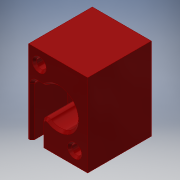
# Autodesk Inventor part: Base
Saved by Autodesk Inventor 2019 (Build 230136000, 136)
## iProperties
Created: 2021-01-03
Part Number: Base
Material: ABS Plastic
Document SubType Name: Modeling
Designer: Sam
Density: 1.06 g/cm^3
Appearance: Red
Author: Sam
Autodesk Inventor part; units mm, degrees
ref_plane "YZ Plane" through (0, 0, 0) normal (1, 0, 0) x (0, 1, 0)
ref_plane "XZ Plane" through (0, 0, 0) normal (0, 1, 0) x (-1, 0, 0)
ref_plane "XY Plane" through (0, 0, 0) normal (0, 0, 1) x (1, 0, 0)
sketch "Sketch1" plane through (0, 0, 0) normal (0, 0, 1) x (1, 0, 0)
  line L0 (12.5, 17.5) -> (-12.5, 17.5)
  line L1 (-12.5, 17.5) -> (-12.5, -17.5)
  line L2 (-12.5, -17.5) -> (12.5, -17.5)
  line L3 (12.5, -17.5) -> (12.5, 17.5)
  point P0 (0, 0)
  point P1 (12.5, 0)
  dimension "d0" = 25
  dimension "d1" = 35
  dimension "d16" = 12.5
  constraints: 8 end point, 2 parallel, 1 horizontal, 1 horizontal alignment, 1 midpoint, 1 perpendicular
  measures "d0" distance of L1.end L2.end
  measures "d1" distance of L2.end L0.start
  measures "d16" distance from line of point (0, 0) L3
extrude "Extrusion1" add sketch "Sketch1" along normal blind 12
sketch "Sketch2" plane through (0, 0, 12) normal (0, 0, 1) x (1, 0, 0)
  circle A0 centre (0, 0) radius 3.05
  dimension "d4" = 6.1
  constraints: 1 centre point, 1 coincident
  measures "d4" diameter of A0
extrude "Extrusion2" cut sketch "Sketch2" against normal up to next
sketch "Sketch4" plane through (0, 0, 12) normal (0, 0, 1) x (1, 0, 0)
  circle A0 centre (0, 0) radius 3.05 projected
  arc A1 (-7, -3.0859) -> (-5.7899, 5) centre (0, 0) ccw
  line L0 (-5.7899, 5) -> (-11, 5)
  line L1 (-11, 5) -> (-11, -17.5)
  line L2 (-12.5, -17.5) -> (12.5, -17.5) projected
  line L3 (-7, -3.0859) -> (-7, -17.5)
  circle A2 centre (0, 0) radius 3.05 projected
  line L4 (12.5, 17.5) -> (-12.5, 17.5) projected
  line L5 (-12.5, 17.5) -> (-12.5, -17.5) projected
  line L6 (-12.5, -17.5) -> (12.5, -17.5) projected
  line L7 (12.5, -17.5) -> (12.5, 17.5) projected
  dimension "d9" = 15.3
  dimension "d10" = 11
  dimension "d11" = 7
  dimension "d12" = 5
  constraints: 6 end point, 2 point on circle, 2 point on line, 1 centre point, 1 coincident, 1 horizontal, 1 parallel, 1 perpendicular
  measures "d9" diameter of A1
  measures "d10" distance from line of point (0, 0) L1
  measures "d11" distance from line of point (0, 0) L3
  measures "d12" distance from line of point (0, 0) L0
extrude "Extrusion3" add sketch "Sketch4" along normal blind 15 contours A1 L0 L1 L2 L5 L4 L7 L3
fillet "Fillet1" radius 2 3 edges at (-7, -3.0859, 19.5) (-5.7899, 5, 19.5) (-11, 5, 19.5)
sketch "Sketch5" plane through (0, 0, 27) normal (0, 0, 1) x (1, 0, 0)
  point P0 (0, 0)
  point P1 (-8, 12)
  point P2 (7, -12)
  dimension "d17" = 7
  dimension "d18" = 12
  dimension "d19" = 12
  dimension "d20" = 8
  measures "d17" horizontal distance of point (7, -12) point (0, 0)
  measures "d18" vertical distance of point (0, 0) point (7, -12)
  measures "d19" vertical distance of point (0, 0) point (-8, 12)
  measures "d20" horizontal distance of point (0, 0) point (-8, 12)
hole "Hole1" at (-8, 12, 27) at (7, -12, 27) direction (0, 0, -1) diameter 4.2 depth 8 tip angle 118 countersink diameter 6 countersink angle 90
chamfer "Chamfer1" distance 1 angle 45 6 edges at (7.606, 0.819, 27) (-5.9817, -6.5111, 27) (-7, -12.8768, 27) (-5.9014, 5.1424, 27) (-7.8212, 5, 27) (-11, -7.25, 27)
body "Solid1"
